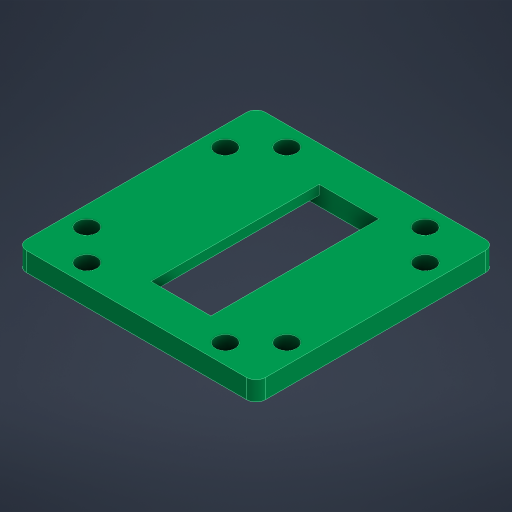
# Autodesk Inventor part: Lens Top Light Cover
Saved by Autodesk Inventor 2023.4 (Build 274418000, 418)
## iProperties
Created: 2024-07-23
Part Number: Lens Top Light Cover
Material: Generic
Document SubType Name: Modeling
Designer: xSibe
Density: 1 g/cm^3
Appearance: Plastic Dark Green
Author: xSibe
Autodesk Inventor part; units mm, degrees
ref_plane "YZ Plane" through (0, 0, 0) normal (1, 0, 0) x (0, 1, 0)
ref_plane "XZ Plane" through (0, 0, 0) normal (0, 1, 0) x (-1, 0, 0)
sketch "Sketch1" plane through (0, 0, 0) normal (0, 1, 0) x (-1, 0, 0)
  line L0 (-155.225, -15) -> (-155.225, 15) projected
  line L1 (-155.225, 15) -> (-147.725, 15) projected
  line L2 (-147.725, 15) -> (-147.725, -15) projected
  line L3 (-147.725, -15) -> (-155.225, -15) projected
  circle A0 centre (-171.5, -21.9) radius 1.875 projected
  circle A1 centre (-127.7, 21.9) radius 1.875 projected
  circle A2 centre (-127.7, -21.9) radius 1.875 projected
  circle A3 centre (-171.5, 21.9) radius 1.875 projected
  circle A4 centre (-135.2, 20.8) radius 2.0734 projected
  circle A5 centre (-164, -20.8) radius 2.0734 projected
  circle A6 centre (-135.2, -20.8) radius 2.0734 projected
  circle A7 centre (-128.8, -14.4) radius 2.0734 projected
  circle A8 centre (-128.8, 14.4) radius 2.0734 projected
  circle A9 centre (-164, 20.8) radius 2.0734 projected
  circle A10 centre (-170.4, -14.4) radius 2.0734 projected
  circle A11 centre (-170.4, 14.4) radius 2.0734 projected
  line L4 (-172.5, 24.875) -> (-126.7, 24.875) projected
  arc A12 (-172.5, 24.875) -> (-174.475, 22.9) centre (-172.5, 22.9) ccw projected
  line L5 (-174.475, -22.9) -> (-174.475, 22.9) projected
  arc A13 (-174.475, -22.9) -> (-172.5, -24.875) centre (-172.5, -22.9) ccw projected
  line L6 (-126.7, -24.875) -> (-172.5, -24.875) projected
  arc A14 (-126.7, -24.875) -> (-124.725, -22.9) centre (-126.7, -22.9) ccw projected
  line L7 (-124.725, 22.9) -> (-124.725, -22.9) projected
  arc A15 (-124.725, 22.9) -> (-126.7, 24.875) centre (-126.7, 22.9) ccw projected
  point P0 (0, 0)
ref_plane "Work Plane1" through (124.725, 49.8, -24.875) normal (0, 1, 0) x (0, 0, 1)
extrude "Extrusion1" add sketch "Sketch1" along normal blind 4 from surface at 49.8 contours A0 | A1 | A2 | A3 | L4 A15 L7 A14 L6 A13 L5 A12
sketch "Sketch2" plane through (126.7, 53.8, -24.875) normal (0, 1, 0) x (1, 0, 0)
  line L0 (28.525, -9.875) -> (21.025, -9.875) projected
  line L1 (28.525, -39.875) -> (28.525, -9.875) projected
  line L2 (21.025, -39.875) -> (28.525, -39.875) projected
  line L3 (21.025, -9.875) -> (21.025, -39.875) projected
  circle A0 centre (8.5, -45.675) radius 2.0734 projected
  circle A1 centre (37.3, -4.075) radius 2.0734 projected
  circle A2 centre (8.5, -4.075) radius 2.0734 projected
  circle A3 centre (2.1, -10.475) radius 2.0734 projected
  circle A4 centre (2.1, -39.275) radius 2.0734 projected
  circle A5 centre (37.3, -45.675) radius 2.0734 projected
  circle A6 centre (43.7, -10.475) radius 2.0734 projected
  circle A7 centre (43.7, -39.275) radius 2.0734 projected
  arc A8 (47.775, -1.975) -> (45.8, 0) centre (45.8, -1.975) ccw projected
  line L4 (0, 0) -> (45.8, 0) projected
  arc A9 (0, 0) -> (-1.975, -1.975) centre (0, -1.975) ccw projected
  line L5 (-1.975, -47.775) -> (-1.975, -1.975) projected
  arc A10 (-1.975, -47.775) -> (0, -49.75) centre (0, -47.775) ccw projected
  line L6 (45.8, -49.75) -> (0, -49.75) projected
  arc A11 (45.8, -49.75) -> (47.775, -47.775) centre (45.8, -47.775) ccw projected
  line L7 (47.775, -1.975) -> (47.775, -47.775) projected
  line L8 (18.525, -42.375) -> (31.025, -42.375)
  line L9 (31.025, -42.375) -> (31.025, -7.375)
  line L10 (31.025, -7.375) -> (18.525, -7.375)
  line L11 (18.525, -7.375) -> (18.525, -42.375)
  line L12 (45.8, 0) -> (50.05, 0)
  line L13 (50.05, 0) -> (50.05, -49.75)
  line L14 (50.05, -49.75) -> (45.8, -49.75)
  line L15 (45.8, -49.75) -> (45.8, 0)
  line L16 (50.05, -49.75) -> (47.925, -49.75)
  line L17 (47.925, -49.75) -> (47.925, 0)
  line L18 (47.925, 0) -> (50.05, 0)
  line L19 (50.05, 0) -> (50.05, -49.75)
  arc A12 (45.8, -49.875) -> (47.9, -47.775) centre (45.8, -47.775) ccw
  line L20 (45.8, -49.875) -> (0, -49.875)
  arc A13 (-2.1, -47.775) -> (0, -49.875) centre (0, -47.775) ccw
  line L21 (-2.1, -47.775) -> (-2.1, -1.975)
  arc A14 (0, 0.125) -> (-2.1, -1.975) centre (0, -1.975) ccw
  line L22 (0, 0.125) -> (45.8, 0.125)
  arc A15 (47.9, -1.975) -> (45.8, 0.125) centre (45.8, -1.975) ccw
  line L23 (47.9, -1.975) -> (47.9, -47.775)
  line L24 (18.525, -42.375) -> (11.025, -42.375)
  line L25 (11.025, -42.375) -> (11.025, -7.375)
  line L26 (11.025, -7.375) -> (18.525, -7.375)
  line L27 (18.525, -7.375) -> (18.525, -42.375)
  line L28 (31.025, -42.375) -> (38.525, -42.375)
  line L29 (38.525, -42.375) -> (38.525, -7.375)
  line L30 (38.525, -7.375) -> (31.025, -7.375)
  line L31 (31.025, -7.375) -> (31.025, -42.375)
  point P0 (-126.7, -24.875)
  point P1 (47.925, -49.75)
  point P2 (46.5137, -49.75)
  point P3 (46.5137, 0)
  point P4 (31.025, -7.375)
  point P5 (18.525, -7.375)
  dimension "d2" = 2.5
  dimension "d3" = 4.25
  dimension "d4" = 2.125
  dimension "d15" = 0.125
  dimension "d16" = 7.5
  dimension "d17" = 7.5
  constraints: 48 end point, 8 parallel, 8 point on circle, 4 centre point, 4 horizontal, 4 perpendicular, 1 collinear, 1 midpoint, 1 point on line, 10 other
  measures "d2" distance between parallel lines of L3 L11
  measures "d3" distance of L6.start L13.end
  measures "d4" distance of L17.end L18.end
  measures "d15" radial gap between concentric circles of A11 A12
  measures "d16" distance of L25.end L26.end
  measures "d17" distance of L30.end L29.end
extrude "Extrusion2" cut sketch "Sketch2" against normal up to surface (4 mm away) contours L11 L10 L9 L8
extrude "Extrusion3" [suppressed]
extrude "Extrusion4" [suppressed]
fillet "Fillet1" [suppressed]
sketch "Sketch3" plane through (176.75, 51.8, 22.875) normal (1, 0, 0) x (0, 0, -1)
  line L0 (7.875, -21.425) -> (7.875, -28.925) projected
  line L1 (7.875, -28.925) -> (37.875, -28.925) projected
  line L2 (37.875, -28.925) -> (37.875, -21.425) projected
  line L3 (37.875, -21.425) -> (7.875, -21.425) projected
  line L4 (5.825, -9.7) -> (39.925, -9.7) projected
  line L5 (39.925, -44.1) -> (39.925, -9.7) projected
  line L6 (5.825, -44.1) -> (39.925, -44.1) projected
  line L7 (5.825, -9.7) -> (5.825, -44.1) projected
  line L8 (2.875, -16.425) -> (2.875, -33.925)
  line L9 (2.875, -33.925) -> (42.875, -33.925)
  line L10 (42.875, -33.925) -> (42.875, -16.425)
  line L11 (42.875, -16.425) -> (2.875, -16.425)
  point P0 (22.875, -51.8)
  dimension "d12" = 5
  constraints: 8 end point, 3 other
  measures "d12" distance between parallel lines of L3 L11
extrude "Extrusion5" [suppressed]
extrude "Extrusion6" cut sketch "Sketch2" along normal blind 2 from surface at -4 contours L24 L25 L26 L11 | L9 L30 L29 L28
body "Solid1"
